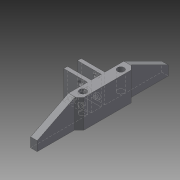
# Autodesk Inventor part: Col support beam
Saved by Autodesk Inventor 2015 (Build 190159000, 159)
## iProperties
Created: 2019-01-12
Part Number: Col support beam
Material: Generic
Document SubType Name: Modeling
Designer: Toby
Density: 1 g/cm^3
Appearance: Default
Author: Toby
Autodesk Inventor part; units mm, degrees
ref_plane "YZ Plane" through (0, 0, 0) normal (1, 0, 0) x (0, 1, 0)
ref_plane "XZ Plane" through (0, 0, 0) normal (0, 1, 0) x (-1, 0, 0)
ref_plane "XY Plane" through (0, 0, 0) normal (0, 0, 1) x (1, 0, 0)
sketch "Sketch1" plane through (0, 0, 0) normal (0, 0, 1) x (1, 0, 0)
  line L0 (14.8889, 11.5915) -> (26.8889, 11.5915)
  line L1 (26.8889, 11.5915) -> (26.8889, -6.9085)
  line L2 (26.8889, -6.9085) -> (14.8889, -6.9085)
  line L3 (14.8889, -6.9085) -> (14.8889, 11.5915)
  line L4 (14.8889, 11.5915) -> (-10.1111, 11.5915)
  line L5 (-10.1111, 11.5915) -> (-10.1111, 7.5915)
  line L6 (-10.1111, 7.5915) -> (14.8889, 7.5915)
  line L7 (14.8889, 7.5915) -> (14.8889, 11.5915)
  line L8 (14.8889, -6.9085) -> (-10.1111, -6.9085)
  line L9 (-10.1111, -6.9085) -> (-10.1111, -2.9085)
  line L10 (-10.1111, -2.9085) -> (14.8889, -2.9085)
  line L11 (14.8889, -2.9085) -> (14.8889, -6.9085)
  point P0 (0, 0)
  dimension "d0" = 10.5
  dimension "d1" = 4
  dimension "d2" = 4
  dimension "d3" = 12
  dimension "d4" = 25
  constraints: 24 end point, 6 parallel, 3 horizontal, 3 perpendicular, 1 point on line
  measures "d0" distance between parallel lines of L10 L6
  measures "d1" distance between parallel lines of L6 L4
  measures "d2" distance between parallel lines of L8 L10
  measures "d3" distance between parallel lines of L1 L3
  measures "d4" distance between parallel lines of L3 L5
extrude "Extrusion1" add sketch "Sketch1" along normal blind 30
sketch "Sketch2" plane through (-10.1111, -6.9085, 0) normal (0, -1, 0) x (1, 0, 0)
  line L0 (0, 30) -> (37, 30) projected
  line L1 (0, 0) -> (37, 0) projected
  line L2 (25, 0) -> (25, 30) projected
  point P0 (10.1111, 0)
  point P1 (18, 25)
  point P2 (18, 5)
  point P3 (8, 5)
  dimension "d7" = 5
  dimension "d8" = 5
  dimension "d9" = 5
  dimension "d10" = 10
  dimension "d11" = 0
  dimension "d12" = 7
  measures "d7" distance from line of L0 point (18, 25)
  measures "d8" distance from line of L1 point (18, 5)
  measures "d9" distance from line of L1 point (8, 5)
  measures "d10" distance of point (18, 5) point (8, 5)
  measures "d11" horizontal distance of point (18, 5) point (18, 25)
  measures "d12" distance from line of L2 point (18, 25)
hole "Hole1" at (7.8889, -6.9085, 25) at (7.8889, -6.9085, 5) at (-2.1111, -6.9085, 5) direction (0, 1, 0) diameter 3 depth 8 tip angle 118 countersink diameter 6 countersink angle 90
sketch "Sketch3" plane through (-10.1111, 11.5915, 0) normal (0, 1, 0) x (1, 0, 0)
  circle A0 centre (18, -25) radius 1.5 projected
  circle A1 centre (18, -5) radius 1.5 projected
  circle A2 centre (8, -5) radius 1.5 projected
  point P0 (10.1111, 0)
  constraints: 3 coincident
hole "Hole2" at (7.8889, 11.5915, 25) at (7.8889, 11.5915, 5) at (-2.1111, 11.5915, 5) direction (0, -1, 0) diameter 3 depth 10 tip angle 118 counterbore diameter 6 counterbore depth 2
chamfer "Chamfer1" distance 5 angle 45 1 edges at (26.8889, 2.3415, 0)
sketch "Sketch4" plane through (0, 0, 30) normal (0, 0, 1) x (1, 0, 0)
  line L0 (21.8889, 11.5915) -> (14.8889, 11.5915)
  line L1 (14.8889, 11.5915) -> (14.8889, 71.5915)
  line L2 (14.8889, 71.5915) -> (21.8889, 71.5915)
  line L3 (21.8889, 71.5915) -> (21.8889, 11.5915)
  line L4 (-10.1111, -6.9085) -> (21.8889, -6.9085) projected
  line L5 (14.8889, -6.9085) -> (21.8889, -6.9085)
  line L6 (21.8889, -6.9085) -> (21.8889, -66.9085)
  line L7 (21.8889, -66.9085) -> (14.8889, -66.9085)
  line L8 (14.8889, -66.9085) -> (14.8889, -6.9085)
  line L9 (14.8889, 7.5915) -> (14.8889, -2.9085) projected
  point P0 (0, 0)
  dimension "d30" = 60
  dimension "d31" = 60
  constraints: 16 end point, 4 parallel, 3 point on line, 2 horizontal, 2 perpendicular, 1 collinear
  measures "d30" distance between parallel lines of L0 L2
  measures "d31" distance between parallel lines of L4 L7
extrude "Extrusion2" add sketch "Sketch4" against normal blind 30
sketch "Sketch5" plane through (0, 0, 30) normal (0, 0, 1) x (1, 0, 0)
  line L0 (14.8889, 7.5915) -> (14.8889, -2.9085) projected
  line L1 (14.8889, 2.3415) -> (26.8889, 2.3415)
  line L2 (26.8889, 2.3415) -> (26.8889, 27.3415)
  line L3 (26.8889, 27.3415) -> (14.8889, 27.3415)
  line L4 (14.8889, 27.3415) -> (14.8889, 2.3415)
  line L5 (14.8889, 2.3415) -> (26.8889, 2.3415)
  line L6 (26.8889, 2.3415) -> (26.8889, -22.6585)
  line L7 (26.8889, -22.6585) -> (14.8889, -22.6585)
  line L8 (14.8889, -22.6585) -> (14.8889, 2.3415)
  line L9 (26.8889, -6.9085) -> (26.8889, 11.5915) projected
  point P0 (0, 0)
  dimension "d34" = 25
  dimension "d35" = 25
  constraints: 16 end point, 4 parallel, 2 horizontal, 2 perpendicular, 1 collinear, 1 midpoint, 1 point on line
  measures "d34" distance between parallel lines of L1 L3
  measures "d35" distance between parallel lines of L1 L7
extrude "Extrusion3" add sketch "Sketch5" against normal blind 30
sketch "Sketch6" plane through (0, 0, 30) normal (0, 0, 1) x (1, 0, 0)
  line L0 (26.8889, -22.6585) -> (26.8889, 27.3415) projected
  line L1 (26.8889, 27.3415) -> (21.8889, 27.3415) projected
  circle A0 centre (20.8889, 22.3415) radius 3.5
  circle A1 centre (20.8889, -17.6585) radius 3.5
  point P0 (0, 0)
  dimension "d38" = 40
  dimension "d39" = 6
  dimension "d40" = 6
  dimension "d41" = 5
  dimension "d42" = 7
  dimension "d43" = 7
  constraints: 2 centre point, 2 coincident
  measures "d38" distance of point (20.889, -17.658) point (20.889, 22.342)
  measures "d39" distance from line of L0 point (20.889, 22.342)
  measures "d40" distance from line of L0 point (20.889, -17.658)
  measures "d41" distance from line of L1 point (20.889, 22.342)
  measures "d42" diameter of A0
  measures "d43" diameter of A1
extrude "Extrusion4" cut sketch "Sketch6" against normal blind 20
chamfer "Chamfer2" distance 5 angle 45 2 edges at (21.8889, -22.6585, 15) (21.8889, 27.3415, 15)
chamfer "Chamfer3" distance 20 distance2 40 1 edges at (18.3889, -66.9085, 30) measured on face at (18.3889, -66.9085, 29.5)
chamfer "Chamfer4" distance 20 distance2 40 1 edges at (18.3889, 71.5915, 30) measured on face at (18.3889, 71.5915, 29.5)
body "Solid1"
